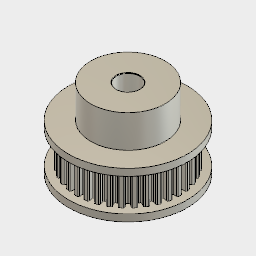
1253 Aluminum Timing Pulley (Autodesk Fusion 360 design; units mm, degrees)
Autodesk Fusion 360 part; units mm, degrees
sketch "Sketch1" plane through (0, 0, 0) normal (0, 1, 0) x (1, 0, 0)
  circle A0 centre (0, 0) radius 12.75
  dimension "d1" = 25.5
  measures "d1" diameter of A0
extrude "Extrude1" add sketch "Sketch1" along normal blind 1.5
sketch "Sketch2" plane through (0, 1.5, 0) normal (0, 1, 0) x (-1, 0, 0)
  circle A0 centre (0, 0) radius 12.75
  circle A1 centre (0, 0) radius 10
  dimension "d4" = 20
  measures "d4" diameter of A1
extrude "Extrude2" add sketch "Sketch2" along normal blind 7 contours A1
sketch "Sketch3" plane through (0, 8.5, 0) normal (0, 1, 0) x (-1, 0, 0)
  circle A0 centre (0, 0) radius 10
  circle A1 centre (0, 0) radius 11.2
  line L0 (0, 0) -> (0, -11.2)
  circle A2 centre (0, 0) radius 10
  line L1 (0.5, -9.9875) -> (0.5, -11.1888)
  line L2 (-0.5, -9.9875) -> (-0.5, -11.1888)
  dimension "d8" = 11.2
  dimension "d9" = 1
  measures "d8" radius of A1
  measures "d9" distance of L1 L2
extrude "Extrude3" add sketch "Sketch3" against normal up to surface (7 mm away) contours A0 A1 L0 A2 L2 | A0 A1 L0 A2 L1
fillet "Fillet1" radius 0.25 4 edges at (0.5, 5, -11.1888) (-0.5, 5, -11.1888) (0.5, 5, -9.9875) (-0.5, 5, -9.9875)
pattern_circular "C-Pattern1" count 36 over 360 about axis through (0, 8.5, 0) along (0, 1, 0) of "Extrude3", "Fillet1"
ref_plane "WorkPlane1" through (0, 5, 0) normal (0, 1, 0) x (-1, 0, 0)
mirror "Mirror1" about plane through (0, 5, 0) normal (0, 1, 0) of "Extrude1"
sketch "Sketch4" plane through (0, 10, 0) normal (0, 1, 0) x (-1, 0, 0)
  circle A0 centre (0, 0) radius 12.75
  circle A1 centre (0, 0) radius 8
  dimension "d16" = 16
  measures "d16" diameter of A1
extrude "Extrude4" add sketch "Sketch4" along normal blind 7 contours A1
sketch "Sketch5" plane through (0, 17, 0) normal (0, 1, 0) x (-1, 0, 0)
  circle A0 centre (0, 0) radius 8
  circle A1 centre (0, 0) radius 2.5
  dimension "d19" = 5
  measures "d19" diameter of A1
extrude "Extrude5" cut sketch "Sketch5" against normal up to surface (17 mm away) contours A1
chamfer "Chamfer1" distance 0.1 angle 45 2 edges at (2.3308, 17, 0.904) (2.3308, 0, -0.904)
